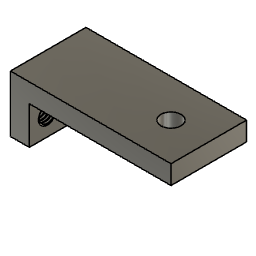
배터리 박스 브라켓 (Autodesk Fusion 360 design; units mm, degrees)
Autodesk Fusion 360 part; units mm, degrees
sketch "스케치1" plane through (0, 0, 0) normal (1, 0, 0) x (0, 1, 0)
  line L0 (0, 0) -> (20, 0)
  line L1 (20, 0) -> (20, 15)
  line L2 (20, 15) -> (0, 15)
  line L3 (0, 15) -> (0, 0)
  line L4 (0, 15) -> (20, 15)
  line L5 (20, 15) -> (20, 10)
  line L6 (20, 10) -> (0, 10)
  line L7 (0, 10) -> (0, 15)
  circle A0 centre (5, 5) radius 2.65
  circle A1 centre (15, 5) radius 2.65
  dimension "d1" = 20
  dimension "d2" = 15
  dimension "d3" = 5
  dimension "d4" = 5.3
  dimension "d5" = 5.3
  constraint horizontal L0
  constraint vertical L1
  constraint horizontal L2
  constraint vertical L3
  constraint coincident L0.start L3.end
  constraint horizontal L4
  constraint vertical L5
  constraint horizontal L6
  constraint vertical L7
  measures "d1" distance of L0.start L0.end
  measures "d2" distance of L0.start L2.end
  measures "d3" distance of L2.end L6.end
  measures "d4" diameter of A0
  measures "d5" diameter of A1
extrude "돌출1" add sketch "스케치1" along normal blind 5 contours L0 L1 L3 L6
extrude "돌출2" add sketch "스케치1" along normal blind 42.5 contours L1 L2 L3 L4 L5 L6 L7
sketch "스케치2" plane through (0, 0, 15) normal (0, 0, 1) x (-1, 0, 0)
  line L0 (0, -20) -> (0, 0)
  line L1 (0, 0) -> (-42.5, 0)
  line L2 (-42.5, 0) -> (-42.5, -20)
  line L3 (-42.5, -20) -> (0, -20)
  line L4 (-42.5, -20) -> (-22.5, -20)
  line L5 (-22.5, -20) -> (-22.5, 0)
  line L6 (-22.5, 0) -> (-42.5, 0)
  line L7 (-42.5, 0) -> (-42.5, -20)
  circle A0 centre (-32.5, -10) radius 2.65
  dimension "d10" = 20
  dimension "d11" = 20
  dimension "d17" = 5.3
  constraint horizontal L4
  constraint vertical L5
  constraint horizontal L6
  constraint vertical L7
  constraint coincident L2.end L3.start
  measures "d10" distance of L2.end L4.end
  measures "d11" distance of L2.end L1.end
  measures "d17" diameter of A0
extrude "돌출3" cut sketch "스케치2" against normal blind 13 contours A0
thread "나사산1" "ISO Metric profile 5.0 M5x0.8 6H" major diameter 5.12 minor diameter 4.234 pitch 0.8 angle 60 modelled right hand crest width 0.2219 on face at (3.3333, 7.6467, 4.8679) crest through (0.2, 7.117, 5) on face at (3.3333, 17.6467, 4.8679) crest through (0.2, 17.117, 5)
